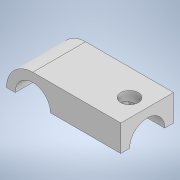
# Autodesk Inventor part: AbrazaderaBarraAscenso2
Saved by Autodesk Inventor 2021 (Build 250183000, 183)
## iProperties
Created: 2021-04-19
Part Number: AbrazaderaBarraAscenso2
Material: Generic
Document SubType Name: Modeling
Designer: GABRIEL LOL
Density: 1 g/cm^3
Appearance: Default
Author: GABRIEL LOL
Autodesk Inventor part; units mm, degrees
ref_plane "YZ Plane" through (0, 0, 0) normal (1, 0, 0) x (0, 1, 0)
ref_plane "XZ Plane" through (0, 0, 0) normal (0, 1, 0) x (-1, 0, 0)
ref_plane "XY Plane" through (0, 0, 0) normal (0, 0, 1) x (1, 0, 0)
sketch "Sketch1" plane through (0, 0, 0) normal (0, 0, 1) x (1, 0, 0)
  circle A0 centre (0, 0) radius 10
  circle A1 centre (0, 0) radius 15
  line L0 (0, 15) -> (50, 15)
  line L1 (50, 15) -> (50, -15)
  line L2 (0, -15) -> (50, -15)
  line L3 (-15, 0) -> (50, 0)
  point P0 (-10, 0)
  point P1 (10, 0)
  dimension "d0" = 20
  dimension "d1" = 30
  dimension "d2" = 50
  constraints: 9 end point, 3 point on circle, 2 centre point, 2 coincident, 2 horizontal, 1 midpoint, 1 perpendicular, 1 tangent
  measures "d0" diameter of A0
  measures "d1" diameter of A1
  measures "d2" distance of L0.start L0.end
extrude "Extrusion1" add sketch "Sketch1" along normal blind 30 contours A0 L3 A1 | A1 L0 L1 L3 picked at (13.208, 1.1126)
sketch "Sketch2" plane through (50, 0, 0) normal (1, 0, 0) x (0, 0, -1)
  line L0 (0, 0) -> (-30, 0) projected
  circle A0 centre (-15, 0) radius 10
  point P0 (-25, 0)
  point P1 (-5, 0)
  dimension "d5" = 20
  constraints: 1 centre point, 1 midpoint
  measures "d5" diameter of A0
extrude "Extrusion2" cut sketch "Sketch2" against normal blind 20 contours L0 A0 picked at (-12.505, 2.2104)
sketch "Sketch3" plane through (0, 15, 0) normal (0, 1, 0) x (1, 0, 0)
  line L0 (50, 0) -> (0, 0) projected
  line L1 (0, 0) -> (0, -30) projected
  line L2 (50, -30) -> (0, -30) projected
  line L3 (50, 0) -> (50, -30) projected
  line L4 (50, -5) -> (50, -25) construction
  circle A0 centre (40, -15) radius 5
  line L5 (30, -5) -> (30, -25) projected
  line L6 (40, -15) -> (30, -15) construction
  dimension "d8" = 10
  dimension "d12" = 10
  constraints: 2 end point, 1 centre point, 1 midpoint
  measures "d8" diameter of A0
  measures "d12" distance of L6.start L6.end
extrude "Extrusion3" cut sketch "Sketch3" against normal blind 10 contours A0
body "Solid1"
